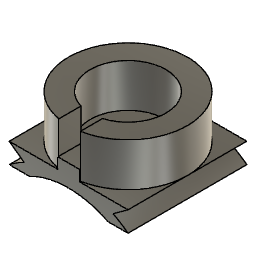
finger_bowden_place_holder (Autodesk Fusion 360 design; units mm, degrees)
Autodesk Fusion 360 part; units mm, degrees
note: some values were not read from the file. Set by a fixed rule: which sketch regions a step uses.
sketch "Esquisse1" plane through (0, 0, 0) normal (0, 0, 1) x (1, 0, 0)
  circle A0 centre (47.4696, 29.6196) radius 5.5
  circle A1 centre (47.4696, 29.6196) radius 3.5
  line L0 (47.4696, 29.6196) -> (47.4696, 24.1196)
  line L1 (46.4696, 26.2655) -> (48.4696, 26.2655)
  line L2 (48.4696, 26.2655) -> (48.4696, 24.1196)
  line L3 (48.4696, 24.1196) -> (46.4696, 24.1196)
  line L4 (46.4696, 24.1196) -> (46.4696, 26.2655)
  dimension "d5" = 7
  dimension "d6" = 2
  dimension "d7" = 1
  constraint concentric A0 A1
  constraint coincident A0.centre A1.centre
  constraint coincident A0 L0.end
  constraint vertical L0
  constraint horizontal L1
  constraint vertical L2
  constraint horizontal L3
  constraint vertical L4
  constraint coincident A1 L1.start
  constraint coincident L0.end L3
  constraint coincident A1 L1.end
  measures "d5" diameter of A1
  measures "d6" distance of A0 A1
  measures "d7" distance of L0 L2
extrude "Extrusion1" add sketch "Esquisse1" along normal blind 4 contours A0 A1 L2 L4
extrude "Extrusion2" add sketch "Esquisse1" along normal blind 1 contours A0 A1 L0 L4 | A0 L3 L4 | A0 L2 L3 | A0 A1 L0 L2
sketch "Esquisse2" plane through (0, 24.1196, 0) normal (0, -1, 0) x (1, 0, 0)
  line L0 (46.4696, 0) -> (48.4696, 0)
  line L1 (48.4696, 0) -> (48.4696, 1)
  line L2 (48.4696, 1) -> (46.4696, 1)
  line L3 (46.4696, 1) -> (46.4696, 0)
  circle A0 centre (47.4696, -9) radius 8
  circle A1 centre (47.4696, -9) radius 9
  line L4 (47.4696, 0) -> (47.4696, -9)
  line L5 (48.4696, 0) -> (46.4696, 0)
  line L6 (43.3465, -1) -> (51.5927, -1)
  line L7 (51.5927, -1) -> (52.9696, 0)
  line L8 (41.9696, 0) -> (43.3465, -1)
  line L9 (47.4696, 0) -> (41.9696, 0)
  line L10 (47.4696, 0) -> (52.9696, 0)
  line L11 (38.9843, -6) -> (55.9549, -6)
  line L12 (41.9696, -1.8761) -> (52.9696, -1.8761)
  dimension "d12" = 1
  dimension "d13" = 16
  dimension "d14" = 5.5
  dimension "d15" = 5.5
  dimension "d16" = 5
  constraint concentric A0 A1
  constraint midpoint L0 L4.start
  constraint perpendicular L0 L4
  constraint coincident A0.centre A1.centre
  constraint tangent A1 L5
  constraint horizontal L6
  constraint tangent A0 L6
  constraint coincident A1 L6.start
  constraint coincident A1 L6.end
  constraint tangent A1 L9
  constraint perpendicular L4 L10
  constraint coincident A1 L11.start
  constraint coincident A1 L11.end
  constraint horizontal L11
  constraint coincident A1 L12.start
  constraint coincident A1 L12.end
  constraint parallel L11 L12
  measures "d12" distance of A0 A1
  measures "d13" diameter of A0
  measures "d14" distance of L4.start L8.start
  measures "d15" distance of L4.start L7.end
  measures "d16" distance of L6 L11
extrude "Extrusion3" add sketch "Esquisse2" against normal blind 11 contours L0 A1 L5 L8 L9 | L0 A1 L5 L7 L10 | A1 L4 L6 | A1 L4 L6 | A0 A1 L6 L12 | A0 A1 L6 L12
